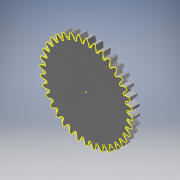
# Autodesk Inventor part: Цилиндрическое зубчатое зацепление2
Saved by Autodesk Inventor 2019 (Build 230136000, 136)
## iProperties
Created: 2020-02-27
Part Number: Цилиндрическое зубчатое зацепление2
Material: Steel
Document SubType Name: Modeling
Designer: Петров Иван
Categories: <?xml version="1.0" encoding="UTF-16"?> <MemberInstance><Categories><FamilyTemplate><FamilyTemplateParameter ValueType="xs:double" Id="1" ObjectReferenceKey="da_z" ObjectType="kUserParameterObject"/><FamilyTemplateParameter ValueType="xs:double" Id="2" ObjectReferenceKey="da_b" ObjectType="kUserParameterObject"/><FamilyTemplateParameter ValueType="xs:double" Id="3" ObjectReferenceKey="da_beta" ObjectType="kUserParameterObject"/><FamilyTemplateParameter ValueType="xs:double" Id="4" ObjectReferenceKey="da_da" ObjectType="kUserParameterObject"/><FamilyTemplateParameter ValueType="xs:double" Id="5" ObjectReferenceKey="da_aw" ObjectType="kUserParameterObject"/><FamilyTemplateParameter ValueType="xs:string" Id="6" ObjectReferenceKey="EAIAABAAAACIAQAAAAAAAIAAAAAAAAAA" ObjectType="83910656" SubObjectId="SurfaceGeometry"/></FamilyTemplate><ParamToTemplateMap><ParamToTemplate CategoryParameter="//CategoryParameter[@InternalName='046C89C9-8512-4d59-83FE-43B91F4F132A']" TemplateParameter="1"/><ParamToTemplate CategoryParameter="//CategoryParameter[@InternalName='2552DF32-E462-4b46-AEBF-C6C7768E72AC']" TemplateParameter="2"/><ParamToTemplate CategoryParameter="//CategoryParameter[@InternalName='C9EE641D-15FC-4fae-A226-E94C4372FDD7']" TemplateParameter="3"/><ParamToTemplate><ParamToTemplate CategoryParameter="//CategoryParameter[@InternalName='00B6519A-459B-49c7-AD84-2E56D39A5744']" ConstantValue="-0.327003"/></ParamToTemplate><ParamToTemplate><ParamToTemplate CategoryParameter="//CategoryParameter[@InternalName='04B31F0E-C7A6-4894-AA32-9629BEFACF47']" ConstantValue="1.000000"/></ParamToTemplate><ParamToTemplate><ParamToTemplate CategoryParameter="//CategoryParameter[@InternalName='43CBEC2E-7847-49e7-A936-2F7889FCB2D9']" ConstantValue="0.250000"/></ParamToTemplate><ParamToTemplate><ParamToTemplate CategoryParameter="//CategoryParameter[@InternalName='B1EFC894-105D-4ebd-86BF-FA20ED196853']" ConstantValue="0.350000"/></ParamToTemplate><ParamToTemplate><ParamToTemplate CategoryParameter="//CategoryParameter[@InternalName='51175063-3D10-4879-93E8-6246FE8B403D']" ConstantValue="2060000000.000000"/></ParamToTemplate><ParamToTemplate><ParamToTemplate CategoryParameter="//CategoryParameter[@InternalName='A3A52E27-4454-46a9-B0BD-C932399B70AF']" ConstantValue="0.300000"/></ParamToTemplate><ParamToTemplate><ParamToTemplate CategoryParameter="//CategoryParameter[@InternalName='91B76062-C214-41d9-B1B9-14D2AB99603D']" ConstantValue="0.225000"/></ParamToTemplate><ParamToTemplate><ParamToTemplate CategoryParameter="//CategoryParameter[@InternalName='374E806E-8B8A-4dda-A9AA-1039D6500AD2']" ConstantValue="4.444444"/></ParamToTemplate><ParamToTemplate><ParamToTemplate CategoryParameter="//CategoryParameter[@InternalName='2D373A89-B862-43d6-8D0B-0CBF12AB9F6C']" ConstantValue="0.523599"/></ParamToTemplate><ParamToTemplate CategoryParameter="//CategoryParameter[@InternalName='37777632-D6A2-4fac-9D53-DB8ACD95C989']" TemplateParameter="4"/><ParamToTemplate CategoryParameter="//CategoryParameter[@InternalName='FD1017F1-B727-4f7e-9707-0F86F1FF9423']" TemplateParameter="5"/><ParamToTemplate><ParamToTemplate CategoryParameter="//CategoryParameter[@InternalName='9E1B4470-B2D3-4ff1-B813-535BB4CDF51A']" ConstantValue="3520000.000000"/></ParamToTemplate><ParamToTemplate><ParamToTemplate CategoryParameter="//CategoryParameter[@InternalName='F8452263-BFF6-458c-9FB1-07C4B99E95CD']" ConstantValue="11400000.000000"/></ParamToTemplate><ParamToTemplate><ParamToTemplate CategoryParameter="//CategoryParameter[@InternalName='3E3BB259-FD49-497f-8171-6EBC954A3479']" ConstantValue="2.000000"/></ParamToTemplate><ParamToTemplate CategoryParameter="//CategoryParameter[@InternalName='27C3BAF2-7550-4e4b-AE2C-0DB134B7D9B7']" TemplateParameter="6"/></ParamToTemplateMap><Category DisplayName="Gear" InternalName="DC85795E-93AB-48d5-8EEE-5A27447B64BD" Mnemonic="Gear"><CategoryParameter DisplayName="z" InternalName="046C89C9-8512-4d59-83FE-43B91F4F132A" Mnemonic="z"/><CategoryParameter DisplayName="b" InternalName="2552DF32-E462-4b46-AEBF-C6C7768E72AC" Mnemonic="b"/><CategoryParameter DisplayName="||b|" InternalName="C9EE641D-15FC-4fae-A226-E94C4372FDD7" Mnemonic="beta"/><CategoryParameter DisplayName="x" InternalName="00B6519A-459B-49c7-AD84-2E56D39A5744" Mnemonic="x"/><CategoryParameter DisplayName="a*" InternalName="04B31F0E-C7A6-4894-AA32-9629BEFACF47" Mnemonic="a"/><CategoryParameter DisplayName="c*" InternalName="43CBEC2E-7847-49e7-A936-2F7889FCB2D9" Mnemonic="c"/><CategoryParameter DisplayName="r|.f|*" InternalName="B1EFC894-105D-4ebd-86BF-FA20ED196853" Mnemonic="rf"/><CategoryParameter DisplayName="E" InternalName="51175063-3D10-4879-93E8-6246FE8B403D" Mnemonic="E"/><CategoryParameter DisplayName="||m|" InternalName="A3A52E27-4454-46a9-B0BD-C932399B70AF" Mnemonic="mi"/><Category DisplayName="SpurGear" InternalName="26C5A22E-A91E-4dfd-A3B3-23CCAFAE1764" Mnemonic="SpurGear"><CategoryParameter DisplayName="m" InternalName="91B76062-C214-41d9-B1B9-14D2AB99603D" Mnemonic="m"/><CategoryParameter DisplayName="P" InternalName="374E806E-8B8A-4dda-A9AA-1039D6500AD2" Mnemonic="PP"/><CategoryParameter DisplayName="||a|" InternalName="2D373A89-B862-43d6-8D0B-0CBF12AB9F6C" Mnemonic="alpha"/><CategoryParameter DisplayName="d|.a|" InternalName="37777632-D6A2-4fac-9D53-DB8ACD95C989" Mnemonic="da"/><CategoryParameter DisplayName="a|.w|" InternalName="FD1017F1-B727-4f7e-9707-0F86F1FF9423" Mnemonic="aw"/><CategoryParameter DisplayName="||s||.Flim|" InternalName="9E1B4470-B2D3-4ff1-B813-535BB4CDF51A" Mnemonic="sFlim"/><CategoryParameter DisplayName="||s||.Hlim|" InternalName="F8452263-BFF6-458c-9FB1-07C4B99E95CD" Mnemonic="sHlim"/><CategoryParameter DisplayName="тип" InternalName="3E3BB259-FD49-497f-8171-6EBC954A3479" Mnemonic="type"/><CategoryParameter DisplayName="PitchDiameter" InternalName="27C3BAF2-7550-4e4b-AE2C-0DB134B7D9B7" Mnemonic="IDS_PITCHDIAM"/></Category></Category></Categories></MemberInstance>
Density: 1 g/cm^3
Appearance: Steel
CustomPartVersion: 1
Author: Петров Иван
Autodesk Inventor part; units mm, degrees
ref_plane "YZ Plane" through (0, 0, 0) normal (1, 0, 0) x (0, 1, 0)
ref_plane "XZ Plane" through (0, 0, 0) normal (0, 1, 0) x (-1, 0, 0)
ref_plane "XY Plane" through (0, 0, 0) normal (0, 0, 1) x (1, 0, 0)
sketch "Sketch1" plane through (0, 0, 0) normal (0, 0, 1) x (1, 0, 0)
  circle A0 centre (0, 0) radius 42
  dimension "d0" = 84
  constraints: 1 centre point
  measures "d0" diameter of A0
extrude "Extrusion1" add sketch "Sketch1" along normal blind 7
ref_plane "Work Plane2" through (0, 0, 3.5) normal (0, 0, 1) x (1, 0, 0)
sketch "Sketch2" plane through (0, 0, 0) normal (0, 0, -1) x (-1, 0, 0)
  circle A0 centre (0, 0) radius 42 projected
  circle A1 centre (0, 0) radius 40
  dimension "d3" = 80
  constraints: 1 centre point, 1 coincident
  measures "d3" diameter of A1
surface extrude "Средний диаметр" sketch "Sketch2" against normal through all shown no curves A1
ref_plane "Work Plane8" through (0, 0, 0) normal (0.9961947, 0.0871557, 0) x (0, 0, 1)
ref_plane "Work Plane9" through (0, 0, 0) normal (1, 0, 0) x (0, 1, 0)
spur gear teeth "Цилиндрическое зубчатое зацепление" teeth 36 pitch diameter 81 tip diameter 84 root diameter 73.9035 face width 7 start plane through (0, 0, 0) normal (0, 0, -1) x (-1, 0, 0)
sketch "Эскиз3" plane through (0, 0, 7) normal (0, 0, 1) x (1, 0, 0)
  arc A0 (-8.1938, 41.193) -> (-8.7829, 35.8928) centre (15.46, 35.881) ccw projected
  arc A1 (-8.7829, 35.8928) -> (-10.3402, 35.4755) centre (0, 0) ccw projected
  arc A2 (-10.3402, 35.4755) -> (-13.5005, 39.7711) centre (-31.3293, 23.3439) ccw projected
  arc A3 (-13.5005, 39.7711) -> (-15.2224, 39.1443) centre (0, 0) ccw projected
  arc A4 (-15.2224, 39.1443) -> (-14.8822, 33.8224) centre (8.9945, 38.0205) ccw projected
  arc A5 (-14.8822, 33.8224) -> (-16.3433, 33.141) centre (0, 0) ccw projected
  arc A6 (-16.3433, 33.141) -> (-20.2015, 36.8225) centre (-34.9069, 17.549) ccw projected
  arc A7 (-20.2015, 36.8225) -> (-21.7885, 35.9063) centre (0, 0) ccw projected
  arc A8 (-21.7885, 35.9063) -> (-20.5293, 30.7243) centre (2.2556, 39.0048) ccw projected
  arc A9 (-20.5293, 30.7243) -> (-21.8499, 29.7995) centre (0, 0) ccw projected
  arc A10 (-21.8499, 29.7995) -> (-26.2888, 32.7551) centre (-37.424, 11.2208) ccw projected
  arc A11 (-26.2888, 32.7551) -> (-27.6925, 31.5773) centre (0, 0) ccw projected
  arc A12 (-27.6925, 31.5773) -> (-25.5526, 26.6926) centre (-4.5518, 38.8039) ccw projected
  arc A13 (-25.5526, 26.6926) -> (-26.6926, 25.5526) centre (0, 0) ccw projected
  arc A14 (-26.6926, 25.5526) -> (-31.5773, 27.6925) centre (-38.8039, 4.5518) ccw projected
  arc A15 (-31.5773, 27.6925) -> (-32.7551, 26.2888) centre (0, 0) ccw projected
  arc A16 (-32.7551, 26.2888) -> (-29.7995, 21.8499) centre (-11.2208, 37.424) ccw projected
  arc A17 (-29.7995, 21.8499) -> (-30.7243, 20.5293) centre (0, 0) ccw projected
  arc A18 (-30.7243, 20.5293) -> (-35.9063, 21.7885) centre (-39.0048, -2.2556) ccw projected
  arc A19 (-35.9063, 21.7885) -> (-36.8225, 20.2015) centre (0, 0) ccw projected
  arc A20 (-36.8225, 20.2015) -> (-33.141, 16.3433) centre (-17.549, 34.9069) ccw projected
  arc A21 (-33.141, 16.3433) -> (-33.8224, 14.8822) centre (0, 0) ccw projected
  arc A22 (-33.8224, 14.8822) -> (-39.1443, 15.2224) centre (-38.0205, -8.9945) ccw projected
  arc A23 (-39.1443, 15.2224) -> (-39.7711, 13.5005) centre (0, 0) ccw projected
  arc A24 (-39.7711, 13.5005) -> (-35.4755, 10.3402) centre (-23.3439, 31.3293) ccw projected
  arc A25 (-35.4755, 10.3402) -> (-35.8928, 8.7829) centre (0, 0) ccw projected
  arc A26 (-35.8928, 8.7829) -> (-41.193, 8.1938) centre (-35.881, -15.46) ccw projected
  arc A27 (-41.193, 8.1938) -> (-41.5112, 6.3892) centre (0, 0) ccw projected
  arc A28 (-41.5112, 6.3892) -> (-36.7321, 4.0228) centre (-28.4295, 26.7997) ccw projected
  arc A29 (-36.7321, 4.0228) -> (-36.8726, 2.4168) centre (0, 0) ccw projected
  arc A30 (-36.8726, 2.4168) -> (-41.99, 0.9162) centre (-32.6513, -21.4558) ccw projected
  arc A31 (-41.99, 0.9162) -> (-41.99, -0.9162) centre (0, 0) ccw projected
  arc A32 (-41.99, -0.9162) -> (-36.8726, -2.4168) centre (-32.6513, 21.4558) ccw projected
  arc A33 (-36.8726, -2.4168) -> (-36.7321, -4.0228) centre (0, 0) ccw projected
  arc A34 (-36.7321, -4.0228) -> (-41.5112, -6.3892) centre (-28.4295, -26.7997) ccw projected
  arc A35 (-41.5112, -6.3892) -> (-41.193, -8.1938) centre (0, 0) ccw projected
  arc A36 (-41.193, -8.1938) -> (-35.8928, -8.7829) centre (-35.881, 15.46) ccw projected
  arc A37 (-35.8928, -8.7829) -> (-35.4755, -10.3402) centre (0, 0) ccw projected
  arc A38 (-35.4755, -10.3402) -> (-39.7711, -13.5005) centre (-23.3439, -31.3293) ccw projected
  arc A39 (-39.7711, -13.5005) -> (-39.1443, -15.2224) centre (0, 0) ccw projected
  arc A40 (-39.1443, -15.2224) -> (-33.8224, -14.8822) centre (-38.0205, 8.9945) ccw projected
  arc A41 (-33.8224, -14.8822) -> (-33.141, -16.3433) centre (0, 0) ccw projected
  arc A42 (-33.141, -16.3433) -> (-36.8225, -20.2015) centre (-17.549, -34.9069) ccw projected
  arc A43 (-36.8225, -20.2015) -> (-35.9063, -21.7885) centre (0, 0) ccw projected
  arc A44 (-35.9063, -21.7885) -> (-30.7243, -20.5293) centre (-39.0048, 2.2556) ccw projected
  arc A45 (-30.7243, -20.5293) -> (-29.7995, -21.8499) centre (0, 0) ccw projected
  arc A46 (-29.7995, -21.8499) -> (-32.7551, -26.2888) centre (-11.2208, -37.424) ccw projected
  arc A47 (-32.7551, -26.2888) -> (-31.5773, -27.6925) centre (0, 0) ccw projected
  arc A48 (-31.5773, -27.6925) -> (-26.6926, -25.5526) centre (-38.8039, -4.5518) ccw projected
  arc A49 (-26.6926, -25.5526) -> (-25.5526, -26.6926) centre (0, 0) ccw projected
  arc A50 (-25.5526, -26.6926) -> (-27.6925, -31.5773) centre (-4.5518, -38.8039) ccw projected
  arc A51 (-27.6925, -31.5773) -> (-26.2888, -32.7551) centre (0, 0) ccw projected
  arc A52 (-26.2888, -32.7551) -> (-21.8499, -29.7995) centre (-37.424, -11.2208) ccw projected
  arc A53 (-21.8499, -29.7995) -> (-20.5293, -30.7243) centre (0, 0) ccw projected
  arc A54 (-20.5293, -30.7243) -> (-21.7885, -35.9063) centre (2.2556, -39.0048) ccw projected
  arc A55 (-21.7885, -35.9063) -> (-20.2015, -36.8225) centre (0, 0) ccw projected
  arc A56 (-20.2015, -36.8225) -> (-16.3433, -33.141) centre (-34.9069, -17.549) ccw projected
  arc A57 (-16.3433, -33.141) -> (-14.8822, -33.8224) centre (0, 0) ccw projected
  arc A58 (-14.8822, -33.8224) -> (-15.2224, -39.1443) centre (8.9945, -38.0205) ccw projected
  arc A59 (-15.2224, -39.1443) -> (-13.5005, -39.7711) centre (0, 0) ccw projected
  arc A60 (-13.5005, -39.7711) -> (-10.3402, -35.4755) centre (-31.3293, -23.3439) ccw projected
  arc A61 (-10.3402, -35.4755) -> (-8.7829, -35.8928) centre (0, 0) ccw projected
  arc A62 (-8.7829, -35.8928) -> (-8.1938, -41.193) centre (15.46, -35.881) ccw projected
  arc A63 (-8.1938, -41.193) -> (-6.3892, -41.5112) centre (0, 0) ccw projected
  arc A64 (-6.3892, -41.5112) -> (-4.0228, -36.7321) centre (-26.7997, -28.4295) ccw projected
  arc A65 (-4.0228, -36.7321) -> (-2.4168, -36.8726) centre (0, 0) ccw projected
  arc A66 (-2.4168, -36.8726) -> (-0.9162, -41.99) centre (21.4558, -32.6513) ccw projected
  arc A67 (-0.9162, -41.99) -> (0.9162, -41.99) centre (0, 0) ccw projected
  arc A68 (0.9162, -41.99) -> (2.4168, -36.8726) centre (-21.4558, -32.6513) ccw projected
  arc A69 (2.4168, -36.8726) -> (4.0228, -36.7321) centre (0, 0) ccw projected
  arc A70 (4.0228, -36.7321) -> (6.3892, -41.5112) centre (26.7997, -28.4295) ccw projected
  arc A71 (6.3892, -41.5112) -> (8.1938, -41.193) centre (0, 0) ccw projected
  arc A72 (8.1938, -41.193) -> (8.7829, -35.8928) centre (-15.46, -35.881) ccw projected
  arc A73 (8.7829, -35.8928) -> (10.3402, -35.4755) centre (0, 0) ccw projected
  arc A74 (10.3402, -35.4755) -> (13.5005, -39.7711) centre (31.3293, -23.3439) ccw projected
  arc A75 (13.5005, -39.7711) -> (15.2224, -39.1443) centre (0, 0) ccw projected
  arc A76 (15.2224, -39.1443) -> (14.8822, -33.8224) centre (-8.9945, -38.0205) ccw projected
  arc A77 (14.8822, -33.8224) -> (16.3433, -33.141) centre (0, 0) ccw projected
  arc A78 (16.3433, -33.141) -> (20.2015, -36.8225) centre (34.9069, -17.549) ccw projected
  arc A79 (20.2015, -36.8225) -> (21.7885, -35.9063) centre (0, 0) ccw projected
  arc A80 (21.7885, -35.9063) -> (20.5293, -30.7243) centre (-2.2556, -39.0048) ccw projected
  arc A81 (20.5293, -30.7243) -> (21.8499, -29.7995) centre (0, 0) ccw projected
  arc A82 (21.8499, -29.7995) -> (26.2888, -32.7551) centre (37.424, -11.2208) ccw projected
  arc A83 (26.2888, -32.7551) -> (27.6925, -31.5773) centre (0, 0) ccw projected
  arc A84 (27.6925, -31.5773) -> (25.5526, -26.6926) centre (4.5518, -38.8039) ccw projected
  arc A85 (25.5526, -26.6926) -> (26.6926, -25.5526) centre (0, 0) ccw projected
  arc A86 (26.6926, -25.5526) -> (31.5773, -27.6925) centre (38.8039, -4.5518) ccw projected
  arc A87 (31.5773, -27.6925) -> (32.7551, -26.2888) centre (0, 0) ccw projected
  arc A88 (32.7551, -26.2888) -> (29.7995, -21.8499) centre (11.2208, -37.424) ccw projected
  arc A89 (29.7995, -21.8499) -> (30.7243, -20.5293) centre (0, 0) ccw projected
  arc A90 (30.7243, -20.5293) -> (35.9063, -21.7885) centre (39.0048, 2.2556) ccw projected
  arc A91 (35.9063, -21.7885) -> (36.8225, -20.2015) centre (0, 0) ccw projected
  arc A92 (36.8225, -20.2015) -> (33.141, -16.3433) centre (17.549, -34.9069) ccw projected
  arc A93 (33.141, -16.3433) -> (33.8224, -14.8822) centre (0, 0) ccw projected
  arc A94 (33.8224, -14.8822) -> (39.1443, -15.2224) centre (38.0205, 8.9945) ccw projected
  arc A95 (39.1443, -15.2224) -> (39.7711, -13.5005) centre (0, 0) ccw projected
  arc A96 (39.7711, -13.5005) -> (35.4755, -10.3402) centre (23.3439, -31.3293) ccw projected
  arc A97 (35.4755, -10.3402) -> (35.8928, -8.7829) centre (0, 0) ccw projected
  arc A98 (35.8928, -8.7829) -> (41.193, -8.1938) centre (35.881, 15.46) ccw projected
  arc A99 (41.193, -8.1938) -> (41.5112, -6.3892) centre (0, 0) ccw projected
  arc A100 (41.5112, -6.3892) -> (36.7321, -4.0228) centre (28.4295, -26.7997) ccw projected
  arc A101 (36.7321, -4.0228) -> (36.8726, -2.4168) centre (0, 0) ccw projected
  arc A102 (36.8726, -2.4168) -> (41.99, -0.9162) centre (32.6513, 21.4558) ccw projected
  arc A103 (41.99, -0.9162) -> (41.99, 0.9162) centre (0, 0) ccw projected
  arc A104 (41.99, 0.9162) -> (36.8726, 2.4168) centre (32.6513, -21.4558) ccw projected
  arc A105 (36.8726, 2.4168) -> (36.7321, 4.0228) centre (0, 0) ccw projected
  arc A106 (36.7321, 4.0228) -> (41.5112, 6.3892) centre (28.4295, 26.7997) ccw projected
  arc A107 (41.5112, 6.3892) -> (41.193, 8.1938) centre (0, 0) ccw projected
  arc A108 (41.193, 8.1938) -> (35.8928, 8.7829) centre (35.881, -15.46) ccw projected
  arc A109 (35.8928, 8.7829) -> (35.4755, 10.3402) centre (0, 0) ccw projected
  arc A110 (35.4755, 10.3402) -> (39.7711, 13.5005) centre (23.3439, 31.3293) ccw projected
  arc A111 (39.7711, 13.5005) -> (39.1443, 15.2224) centre (0, 0) ccw projected
  arc A112 (39.1443, 15.2224) -> (33.8224, 14.8822) centre (38.0205, -8.9945) ccw projected
  arc A113 (33.8224, 14.8822) -> (33.141, 16.3433) centre (0, 0) ccw projected
  arc A114 (33.141, 16.3433) -> (36.8225, 20.2015) centre (17.549, 34.9069) ccw projected
  arc A115 (36.8225, 20.2015) -> (35.9063, 21.7885) centre (0, 0) ccw projected
  arc A116 (35.9063, 21.7885) -> (30.7243, 20.5293) centre (39.0048, -2.2556) ccw projected
  arc A117 (30.7243, 20.5293) -> (29.7995, 21.8499) centre (0, 0) ccw projected
  arc A118 (29.7995, 21.8499) -> (32.7551, 26.2888) centre (11.2208, 37.424) ccw projected
  arc A119 (32.7551, 26.2888) -> (31.5773, 27.6925) centre (0, 0) ccw projected
  arc A120 (31.5773, 27.6925) -> (26.6926, 25.5526) centre (38.8039, 4.5518) ccw projected
  arc A121 (26.6926, 25.5526) -> (25.5526, 26.6926) centre (0, 0) ccw projected
  arc A122 (25.5526, 26.6926) -> (27.6925, 31.5773) centre (4.5518, 38.8039) ccw projected
  arc A123 (27.6925, 31.5773) -> (26.2888, 32.7551) centre (0, 0) ccw projected
  arc A124 (26.2888, 32.7551) -> (21.8499, 29.7995) centre (37.424, 11.2208) ccw projected
  arc A125 (21.8499, 29.7995) -> (20.5293, 30.7243) centre (0, 0) ccw projected
  arc A126 (20.5293, 30.7243) -> (21.7885, 35.9063) centre (-2.2556, 39.0048) ccw projected
  arc A127 (21.7885, 35.9063) -> (20.2015, 36.8225) centre (0, 0) ccw projected
  arc A128 (20.2015, 36.8225) -> (16.3433, 33.141) centre (34.9069, 17.549) ccw projected
  arc A129 (16.3433, 33.141) -> (14.8822, 33.8224) centre (0, 0) ccw projected
  arc A130 (14.8822, 33.8224) -> (15.2224, 39.1443) centre (-8.9945, 38.0205) ccw projected
  arc A131 (15.2224, 39.1443) -> (13.5005, 39.7711) centre (0, 0) ccw projected
  arc A132 (13.5005, 39.7711) -> (10.3402, 35.4755) centre (31.3293, 23.3439) ccw projected
  arc A133 (10.3402, 35.4755) -> (8.7829, 35.8928) centre (0, 0) ccw projected
  arc A134 (8.7829, 35.8928) -> (8.1938, 41.193) centre (-15.46, 35.881) ccw projected
  arc A135 (8.1938, 41.193) -> (6.3892, 41.5112) centre (0, 0) ccw projected
  arc A136 (6.3892, 41.5112) -> (4.0228, 36.7321) centre (26.7997, 28.4295) ccw projected
  arc A137 (4.0228, 36.7321) -> (2.4168, 36.8726) centre (0, 0) ccw projected
  arc A138 (2.4168, 36.8726) -> (0.9162, 41.99) centre (-21.4558, 32.6513) ccw projected
  arc A139 (0.9162, 41.99) -> (-0.9162, 41.99) centre (0, 0) ccw projected
  arc A140 (-0.9162, 41.99) -> (-2.4168, 36.8726) centre (21.4558, 32.6513) ccw projected
  arc A141 (-2.4168, 36.8726) -> (-4.0228, 36.7321) centre (0, 0) ccw projected
  arc A142 (-4.0228, 36.7321) -> (-6.3892, 41.5112) centre (-26.7997, 28.4295) ccw projected
  arc A143 (-6.3892, 41.5112) -> (-8.1938, 41.193) centre (0, 0) ccw projected
equation "\"d0\" = da_da"
equation "\"d1\" = da_b"
equation "\"d3\" = da_dw"
equation "\"da_da\" = 84"
equation "\"da_b\" = 7"
equation "\"da_dw\" = 80"
body "Solid1"
body "Srf1"
